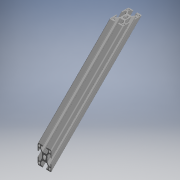
# Autodesk Inventor part: HFBL6-3030-200_b
Saved by Autodesk Inventor 2017.3 (Build 213256000, 256)
## iProperties
Part Number: HFBL6-3030-200_b
Material: Generic
Catalog Web Link: www.cadenas.de
Description: HFBL6_body-Aluminum Frames, Slot Width 8 Series, 30, 50 & 60mm Sections - Fixed Length
Vendor: MISUMI
Document SubType Name: Modeling
Designer: partserver
Manufacturer: MISUMI
Mass: 83.0227 g
Surface Area: 800.031 cm^2
Volume: 83.0227 cm^3
Density: 1 g/cm^3
Appearance: PSOLRGB-192-192-192
Category: PARTsolutions
Company: MISUMI
Title: HFBL6-3030-200_b
Author: Cadenas PARTsolutions
Comments: Aluminum Frames, Slot Width 8 Series, 30, 50 & 60mm Sections - Fixed Length
PSOL_IDENT_0: {$CADENAS_DATA\23d-libs\misumi\metric\38_al_extrusions_blackets\6\hfbl6.prj},182 {VTYP=3D},{NB=HFBL6
PSOL_IDENT_1: -3030-200_b},{LINA=HFBL6-3030-200_b},{NN=HFBL6_body},{DATE=24.04.2017 10:22:41},{GEOMDATE=30.01.2015
PSOL_IDENT_2: 00:00:00},{VERSION=},{LINEID=10},{WBVAR=L,ALT},{WBNUMERIC=L}  {NB=HFBL6-3030-200_b},{LINA=HFBL6-303
PSOL_IDENT_3: 0-200_b},{KT=1},{PN=HFBL6-3030-200},{TP=HFBL6},{NO=3030},{DIM=1.000},{HEIGHT=30},{WIDTH=30},{TYPE=HF
PSOL_IDENT_4: BL6},{MAT=A6N01SS-T5},{ST=Alumite Treatment (No surface treatment on the side cut at 45 degree and
PSOL_IDENT_5: Counterbore type)},{L=200},{LTOL=+/- 0.5},{NOM=8},{DMIN=6.647},{TAPDIST=0},{TAPNO=1},{WHNOHOR=1},{WH
PSOL_IDENT_6: NOVER=1},{WHPOSHOR=0},{WHPOSVER=0},{DHOLEDIAR=0},{DHOLEDIAL=0},{H=15},{ALT4NO=0},{ALT5NO=0},{TAPPOSH
PSOL_IDENT_7: OR=0.000},{TAPPOSVER=0.000},{DRILLLENGTH=200},{AB=CBM6-12},{ABQ=2},{AN=HNTT6-6},{ANQ=2},{ALT=}
NB: HFBL6-3030-200_b
NN: HFBL6_body
NT: Aluminum Frames, Slot Width 8 Series, 30, 50 & 60mm Sections - Fixed Length
NBSYN: $PN._b
LINA: HFBL6-3030-200_b
CATALOG: Misumi
PN: HFBL6-3030-200
NO: 3030
MAT: A6N01SS-T5 Aluminum Alloy
ST: Alumite Treatment (No surface treatment on the side cut at 45 degree and  Counterbore type)
L: 200
AB: CBM6-12
ABQ: 2
AN: HNTT6-6
ANQ: 2
ALT: w/o Set of Applicable Bolt and Nut
SUPPLIER: MISUMI
ARTICLENO: HFBL6-3030-200_b
BOMINFO: HFBL6-3030-200_b
CREATOR: CADENAS GmbH
Autodesk Inventor part; units mm, degrees
sketch "Sketch_1" plane through (0, 0, 0) normal (0, -0.7071, 0.7071) x (1, 0, 0)
  arc A0 (-15, 130.7214) -> (-14.7, 130.4214) centre (-14.7, 130.7214) ccw
  line L0 (-14.7, 130.4214) -> (-13, 130.4214)
  line L1 (-13, 130.4214) -> (-13, 134.6714)
  line L2 (-13, 134.6714) -> (-9.6642, 134.6714)
  line L3 (-9.6642, 134.6714) -> (-6, 131.0072)
  line L4 (-6, 131.0072) -> (-6, 126.941)
  line L5 (-6, 126.941) -> (-5.7, 126.4214)
  line L6 (-5.7, 126.4214) -> (-6, 125.9017)
  line L7 (-6, 125.9017) -> (-6, 121.8356)
  line L8 (-6, 121.8356) -> (-9.6642, 118.1714)
  line L9 (-9.6642, 118.1714) -> (-13, 118.1714)
  line L10 (-13, 118.1714) -> (-13, 122.4214)
  line L11 (-13, 122.4214) -> (-14.7, 122.4214)
  arc A1 (-14.7, 122.4214) -> (-15, 122.1214) centre (-14.7, 122.1214) ccw
  line L12 (-15, 122.1214) -> (-15, 113.4214)
  arc A2 (-15, 113.4214) -> (-13, 111.4214) centre (-13, 113.4214) ccw
  line L13 (-13, 111.4214) -> (-4.3, 111.4214)
  arc A3 (-4.3, 111.4214) -> (-4, 111.7214) centre (-4.3, 111.7214) ccw
  line L14 (-4, 111.7214) -> (-4, 113.4214)
  line L15 (-4, 113.4214) -> (-8.25, 113.4214)
  line L16 (-8.25, 113.4214) -> (-8.25, 116.7572)
  line L17 (-8.25, 116.7572) -> (-4.5858, 120.4214)
  line L18 (-4.5858, 120.4214) -> (-0.5196, 120.4214)
  line L19 (-0.5196, 120.4214) -> (0, 120.7214)
  line L20 (0, 120.7214) -> (0.5196, 120.4214)
  line L21 (0.5196, 120.4214) -> (4.5858, 120.4214)
  line L22 (4.5858, 120.4214) -> (8.25, 116.7572)
  line L23 (8.25, 116.7572) -> (8.25, 113.4214)
  line L24 (8.25, 113.4214) -> (4, 113.4214)
  line L25 (4, 113.4214) -> (4, 111.7214)
  arc A4 (4, 111.7214) -> (4.3, 111.4214) centre (4.3, 111.7214) ccw
  line L26 (4.3, 111.4214) -> (13, 111.4214)
  arc A5 (13, 111.4214) -> (15, 113.4214) centre (13, 113.4214) ccw
  line L27 (15, 113.4214) -> (15, 122.1214)
  arc A6 (15, 122.1214) -> (14.7, 122.4214) centre (14.7, 122.1214) ccw
  line L28 (14.7, 122.4214) -> (13, 122.4214)
  line L29 (13, 122.4214) -> (13, 118.1714)
  line L30 (13, 118.1714) -> (9.6642, 118.1714)
  line L31 (9.6642, 118.1714) -> (6, 121.8356)
  line L32 (6, 121.8356) -> (6, 125.9017)
  line L33 (6, 125.9017) -> (5.7, 126.4214)
  line L34 (5.7, 126.4214) -> (6, 126.941)
  line L35 (6, 126.941) -> (6, 131.0072)
  line L36 (6, 131.0072) -> (9.6642, 134.6714)
  line L37 (9.6642, 134.6714) -> (13, 134.6714)
  line L38 (13, 134.6714) -> (13, 130.4214)
  line L39 (13, 130.4214) -> (14.7, 130.4214)
  arc A7 (14.7, 130.4214) -> (15, 130.7214) centre (14.7, 130.7214) ccw
  line L40 (15, 130.7214) -> (15, 139.4214)
  arc A8 (15, 139.4214) -> (13, 141.4214) centre (13, 139.4214) ccw
  line L41 (13, 141.4214) -> (4.3, 141.4214)
  arc A9 (4.3, 141.4214) -> (4, 141.1214) centre (4.3, 141.1214) ccw
  line L42 (4, 141.1214) -> (4, 139.4214)
  line L43 (4, 139.4214) -> (8.25, 139.4214)
  line L44 (8.25, 139.4214) -> (8.25, 136.0856)
  line L45 (8.25, 136.0856) -> (4.5858, 132.4214)
  line L46 (4.5858, 132.4214) -> (0.5196, 132.4214)
  line L47 (0.5196, 132.4214) -> (0, 132.1214)
  line L48 (0, 132.1214) -> (-0.5196, 132.4214)
  line L49 (-0.5196, 132.4214) -> (-4.5858, 132.4214)
  line L50 (-4.5858, 132.4214) -> (-8.25, 136.0856)
  line L51 (-8.25, 136.0856) -> (-8.25, 139.4214)
  line L52 (-8.25, 139.4214) -> (-4, 139.4214)
  line L53 (-4, 139.4214) -> (-4, 141.1214)
  arc A10 (-4, 141.1214) -> (-4.3, 141.4214) centre (-4.3, 141.1214) ccw
  line L54 (-4.3, 141.4214) -> (-13, 141.4214)
  arc A11 (-13, 141.4214) -> (-15, 139.4214) centre (-13, 139.4214) ccw
  line L55 (-15, 139.4214) -> (-15, 130.7214)
  circle A12 centre (11.625, 138.0464) radius 2.1
  circle A13 centre (11.625, 114.7964) radius 2.1
  circle A14 centre (0, 126.4214) radius 3.4
  circle A15 centre (-11.625, 138.0464) radius 2.1
  circle A16 centre (-11.625, 114.7964) radius 2.1
  constraints: 112 end point, 24 point on circle, 17 centre point
extrude "Extrusion1" add sketch "Sketch_1" along normal mid plane 284.8427
sketch "Sketch_2" plane through (0, 0, 0) normal (0, 0, 1) x (1, 0, 0)
  line L0 (-50, -300) -> (50, -300)
  line L1 (50, -300) -> (50, 0)
  line L2 (50, 0) -> (-50, 0)
  line L3 (-50, 0) -> (-50, -300)
  constraints: 8 end point
extrude "Extrusion2" cut sketch "Sketch_2" along normal blind 400
sketch "Sketch_3" plane through (0, 0, 0) normal (0, 1, 0) x (-1, 0, 0)
  line L0 (50, -300) -> (50, 0)
  line L1 (50, 0) -> (-50, 0)
  line L2 (-50, 0) -> (-50, -300)
  line L3 (-50, -300) -> (50, -300)
  constraints: 8 end point
extrude "Extrusion3" cut sketch "Sketch_3" along normal blind 400
sketch "Sketch_4" plane through (0, 0, 0) normal (1, 0, 0) x (0, 1, 0)
  line L0 (0, 177.25) -> (30, 177.25)
  line L1 (30, 177.25) -> (30, 171.75)
  line L2 (30, 171.75) -> (5, 171.75)
  line L3 (5, 171.75) -> (5, 174)
  line L4 (5, 174) -> (0, 174)
  line L5 (0, 174) -> (0, 177.25)
  line L6 (0, 177.25) -> (30, 177.25)
  constraints: 14 end point
revolve "Revolution1" cut sketch "Sketch_4" angle 360 about axis through (0, 0, 177.25) along (0, -1, 0)
sketch "Sketch_5" plane through (0, 0, 0) normal (1, 0, 0) x (0, 1, 0)
  line L0 (177.25, 0) -> (177.25, 30)
  line L1 (177.25, 30) -> (182.75, 30)
  line L2 (182.75, 30) -> (182.75, 5)
  line L3 (182.75, 5) -> (180.5, 5)
  line L4 (180.5, 5) -> (180.5, 0)
  line L5 (180.5, 0) -> (177.25, 0)
  line L6 (177.25, 0) -> (177.25, 30)
  constraints: 14 end point
revolve "Revolution2" cut sketch "Sketch_5" angle 360 about axis through (0, 177.25, 0) along (0, 0, -1)
ref_plane "bolt1_XY" through (0, 5, 177.25) normal (0, 1, 0) x (1, 0, 0)
ref_plane "bolt1_YZ" through (0, 5, 177.25) normal (1, 0, 0) x (0, 0, -1)
ref_plane "bolt1_ZX" through (0, 5, 177.25) normal (0, 0, -1) x (0, 1, 0)
ref_plane "bolt2_XY" through (0, 177.25, 5) normal (0, 0, 1) x (1, 0, 0)
ref_plane "bolt2_YZ" through (0, 177.25, 5) normal (1, 0, 0) x (0, 1, 0)
ref_plane "bolt2_ZX" through (0, 177.25, 5) normal (0, 1, 0) x (0, 0, 1)
body "Solid1"
